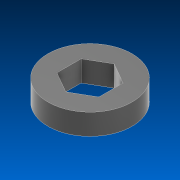
# Autodesk Inventor part: 1_8 Spacer 1_4 Hex Custom
Saved by Autodesk Inventor 2022.2 (Build 262287000, 287)
## iProperties
Created: 2022-01-04
Part Number: 1_8 Spacer 1_4 Hex Custom
Material: PET Plastic
Document SubType Name: Modeling
Designer: omard
Density: 1.541 g/cm^3
Appearance: Smooth - Black
Author: omard
Autodesk Inventor part; units mm, degrees
ref_plane "YZ Plane" through (0, 0, 0) normal (1, 0, 0) x (0, 1, 0)
ref_plane "XZ Plane" through (0, 0, 0) normal (0, 1, 0) x (-1, 0, 0)
ref_plane "XY Plane" through (0, 0, 0) normal (0, 0, 1) x (1, 0, 0)
sketch "Sketch1" plane through (0, 0, 0) normal (0, 1, 0) x (-1, 0, 0)
  line L0 (0, 3.6662) -> (3.175, 1.8331)
  line L1 (3.175, 1.8331) -> (3.175, -1.8331)
  line L2 (3.175, -1.8331) -> (0, -3.6662)
  line L3 (0, -3.6662) -> (-3.175, -1.8331)
  line L4 (-3.175, -1.8331) -> (-3.175, 1.8331)
  line L5 (-3.175, 1.8331) -> (0, 3.6662)
  circle A0 centre (0, 0) radius 6.35
  dimension "d0" = 6.35
  dimension "d1" = 12.7
  constraints: 12 end point, 2 coincident, 1 centre point, 1 vertical, 13 other
  measures "d0" distance between parallel lines of L4 L1
  measures "d1" diameter of A0
extrude "Extrusion1" add sketch "Sketch1" along normal blind 3.175
body "Solid1"
